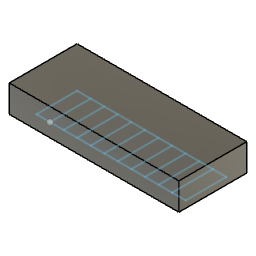
Kerf-test v1 (Autodesk Fusion 360 design; units mm, degrees)
Autodesk Fusion 360 part; units mm, degrees
sketch "Sketch1" plane through (0, 0, 0) normal (0, 0, 1) x (1, 0, 0)
  line L0 (25, 25) -> (150, 25)
  line L1 (150, 25) -> (150, 75)
  line L2 (150, 75) -> (25, 75)
  line L3 (25, 75) -> (25, 25)
  constraint horizontal L0
  constraint vertical L1
  constraint horizontal L2
  constraint vertical L3
extrude "Extrude1" add sketch "Sketch1" along normal blind 20
sketch "Sketch2" plane through (0, 0, 0) normal (0, 0, 1) x (1, 0, 0)
  line L0 (35, 65) -> (135, 65)
  line L1 (135, 65) -> (135, 35)
  line L2 (135, 35) -> (35, 35)
  line L3 (35, 35) -> (35, 65)
  line L4 (45, 65) -> (45, 35)
  line L5 (55, 65) -> (55, 35)
  line L6 (65, 35) -> (65, 65)
  line L7 (75, 65) -> (75, 35)
  line L8 (85, 35) -> (85, 65)
  line L9 (95, 65) -> (95, 35)
  line L10 (105, 35) -> (105, 65)
  line L11 (115, 65) -> (115, 35)
  line L12 (125, 35) -> (125, 65)
  line L13 (135, 35) -> (145, 35)
  line L14 (145, 35) -> (145, 65)
  line L15 (145, 65) -> (135, 65)
  constraint horizontal L0
  constraint vertical L1
  constraint horizontal L2
  constraint vertical L3
  constraint coincident L0 L4.start
  constraint perpendicular L0 L4
  constraint coincident L0 L5.start
  constraint coincident L2 L5.end
  constraint perpendicular L2 L5
  constraint coincident L2 L6.start
  constraint coincident L0 L6.end
  constraint perpendicular L0 L6
  constraint coincident L0 L7.start
  constraint coincident L2 L7.end
  constraint perpendicular L2 L7
  constraint coincident L2 L8.start
  constraint coincident L0 L8.end
  constraint perpendicular L0 L8
  constraint coincident L0 L9.start
  constraint coincident L2 L9.end
  constraint perpendicular L2 L9
  constraint coincident L2 L10.start
  constraint coincident L0 L10.end
  constraint perpendicular L0 L10
  constraint coincident L0 L11.start
  constraint coincident L2 L11.end
  constraint perpendicular L2 L11
  constraint coincident L2 L12.start
  constraint coincident L0 L12.end
  constraint perpendicular L0 L12
  constraint perpendicular L1 L13
  constraint perpendicular L13 L14
  constraint perpendicular L1 L15
